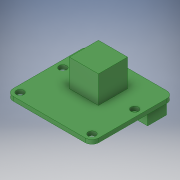
# Autodesk Inventor part: RaspberryPiCamera
Saved by Autodesk Inventor 2019 (Build 230136000, 136)
## iProperties
Created: 2019-04-09
Part Number: RaspberryPiCamera
Material: Generic
Document SubType Name: Modeling
Designer: Epsilon
Density: 1 g/cm^3
Appearance: Smooth - Dark Forest Green
Author: Epsilon
Autodesk Inventor part; units mm, degrees
ref_plane "YZ Plane" through (0, 0, 0) normal (1, 0, 0) x (0, 1, 0)
ref_plane "XZ Plane" through (0, 0, 0) normal (0, 1, 0) x (-1, 0, 0)
ref_plane "XY Plane" through (0, 0, 0) normal (0, 0, 1) x (1, 0, 0)
sketch "Sketch1" plane through (0, 0, 0) normal (0, 1, 0) x (-1, 0, 0)
  line L0 (2, 0) -> (23, 0)
  line L1 (25, -2) -> (25, -21.862)
  line L2 (23, -23.862) -> (2, -23.862)
  line L3 (0, -21.862) -> (0, -2)
  arc A0 (25, -2) -> (23, 0) centre (23, -2) ccw
  arc A1 (23, -23.862) -> (25, -21.862) centre (23, -21.862) ccw
  arc A2 (0, -21.862) -> (2, -23.862) centre (2, -21.862) ccw
  arc A3 (2, 0) -> (0, -2) centre (2, -2) ccw
  line L4 (23, 0) -> (23, -23.862) construction
  line L5 (2, -23.862) -> (2, 0) construction
  line L6 (25, -2) -> (0, -2) construction
  line L7 (0, -14.5) -> (25, -14.5) construction
  circle A4 centre (23, -2) radius 1.1
  circle A5 centre (23, -14.5) radius 1.1
  circle A6 centre (2, -14.5) radius 1.1
  circle A7 centre (2, -2) radius 1.1
  point P0 (0, 0)
  point P1 (25, -23.862)
  point P2 (25, 0)
  point P3 (0, -23.862)
  dimension "d0" = 25
  dimension "d1" = 23.862
  dimension "d2" = 2
  dimension "d3" = 2
  dimension "d4" = 14.5
  dimension "d5" = 2
  dimension "d6" = 2
  dimension "d7" = 2.2
  dimension "d8" = 2.2
  dimension "d9" = 2.2
  dimension "d10" = 2.2
  constraints: 20 point on line, 16 end point, 8 centre point, 8 point on circle, 8 tangent, 6 coincident, 5 perpendicular, 3 equal radius, 2 parallel, 1 horizontal
  measures "d0" distance of point (25, -23.862) point (0, -23.862)
  measures "d1" distance of point (25, 0) point (25, -23.862)
  measures "d2" radius of A0
  measures "d3" distance between parallel lines of L0 L6
  measures "d4" distance between parallel lines of L0 L7
  measures "d5" distance between parallel lines of L3 L5
  measures "d6" distance between parallel lines of L1 L4
  measures "d7" diameter of A4
  measures "d8" diameter of A5
  measures "d9" diameter of A6
  measures "d10" diameter of A7
extrude "Extrusion1" add sketch "Sketch1" along normal blind 1.2
sketch "Sketch2" plane through (0, 1.2, 0) normal (0, 1, 0) x (1, 0, 0)
  line L0 (-25, 21.862) -> (-25, 2) construction
  line L1 (-25, 11.931) -> (0, 11.931) construction
  line L2 (0, 2) -> (0, 21.862) construction
  line L3 (-2, 23.862) -> (-23, 23.862) construction
  line L4 (-12.5, 23.862) -> (-12.5, 0) construction
  line L5 (-23, 0) -> (-2, 0) construction
  line L6 (-16.75, 18.65) -> (-8.25, 18.65)
  line L7 (-8.25, 18.65) -> (-8.25, 10.15)
  line L8 (-8.25, 10.15) -> (-16.75, 10.15)
  line L9 (-16.75, 10.15) -> (-16.75, 18.65)
  line L10 (-16.75, 14.4) -> (-8.25, 14.4) construction
  line L11 (-12.5, 18.65) -> (-12.5, 10.15) construction
  point P0 (0, 0)
  point P1 (-12.5, 14.4)
  dimension "d13" = 8.5
  dimension "d14" = 8.5
  dimension "d15" = 12.5
  dimension "d16" = 9.462
  constraints: 16 end point, 9 midpoint, 2 parallel, 1 horizontal, 1 perpendicular
  measures "d13" distance between parallel lines of L7 L9
  measures "d14" distance between parallel lines of L8 L6
  measures "d15" distance from line of L2 point (-12.5, 14.4)
  measures "d16" distance from line of L3 point (-12.5, 14.4)
extrude "Extrusion2" add sketch "Sketch2" along normal blind 8
sketch "Sketch3" plane through (0, 0, 0) normal (0, -1, 0) x (1, 0, 0)
  line L0 (-2, -23.862) -> (-23, -23.862) projected
  line L1 (-22.9, -23.862) -> (-2.1, -23.862)
  line L2 (-2.1, -23.862) -> (-2.1, -18.362)
  line L3 (-2.1, -18.362) -> (-22.9, -18.362)
  line L4 (-22.9, -18.362) -> (-22.9, -23.862)
  line L5 (-12.5, -18.362) -> (-12.5, -23.862) construction
  point P0 (0, 0)
  dimension "d19" = 20.8
  dimension "d20" = 5.5
  constraints: 10 end point, 3 midpoint, 2 parallel, 1 horizontal, 1 perpendicular, 1 point on line
  measures "d19" distance between parallel lines of L2 L4
  measures "d20" distance between parallel lines of L3 L0
extrude "Extrusion3" add sketch "Sketch3" along normal blind 5
equation "\"d6\" = d5"
equation "\"d7\" = d8"
equation "\"d9\" = d8"
equation "\"d10\" = d8"
body "Solid1"
